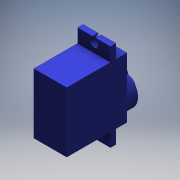
# Autodesk Inventor part: servo
Saved by Autodesk Inventor 2016 (Build 200138000, 138)
## iProperties
Created: 2017-12-28
Part Number: servo
Material: Genérico
Document SubType Name: Sheet Metal
Designer: David
Density: 1 g/cm^3
Sheet Metal Rule: Por defecto_mm
Appearance: Valor por defecto
Author: David
Autodesk Inventor part; units mm, degrees
ref_plane "YZ Plane" through (0, 0, 0) normal (1, 0, 0) x (0, 1, 0)
ref_plane "XZ Plane" through (0, 0, 0) normal (0, 1, 0) x (-1, 0, 0)
ref_plane "XY Plane" through (0, 0, 0) normal (0, 0, 1) x (1, 0, 0)
sketch "Boceto1" plane through (0, 0, 0) normal (0, 1, 0) x (-1, 0, 0)
  line L0 (0, 0) -> (12, 0)
  line L1 (12, 0) -> (12, -11)
  line L2 (12, -11) -> (0, -11)
  line L3 (0, -11) -> (0, 0)
  constraints: 8 end point, 2 parallel, 1 horizontal, 1 perpendicular
extrude "Extrusión1" add sketch "Boceto1" along normal blind 22
sketch "Boceto2" plane through (0, 0, -11) normal (0, 0, -1) x (-1, 0, 0)
  line L0 (12, 22) -> (0, 22) projected
  line L1 (0, 18) -> (12, 18)
  line L2 (0, 16) -> (12, 16)
  line L3 (12, 0) -> (12, 22) projected
  line L4 (0, 18) -> (0, 16)
  line L5 (0, 0) -> (0, 22) projected
  line L6 (12, 18) -> (12, 16)
  constraints: 8 end point, 2 collinear, 2 horizontal, 1 point on line
extrude "Extrusión2" add sketch "Boceto2" along normal blind 5 contours L3 L2 L4 L1
sketch "Boceto3" plane through (-12, 18, -11) normal (0, 1, 0) x (1, 0, 0)
  line L0 (0, 5) -> (12, 5) projected
  arc A0 (5.5, 4.5976) -> (6.5, 4.5976) centre (6, 3.1834) ccw
  line L1 (5.5, 4.5976) -> (5.5, 5)
  line L2 (5.5, 5) -> (6.5, 5)
  line L3 (6.5, 4.5976) -> (6.5, 5)
  point P0 (12, -11)
  constraints: 6 end point, 2 perpendicular, 2 point on circle, 2 point on line, 1 centre point
extrude "Extrusión3" cut sketch "Boceto3" against normal through all
mirror "Simetría1" about plane through (-12, 0, 0) normal (0, 0, 1) of "Extrusión1", "Extrusión2", "Extrusión3"
sketch "Boceto5" plane through (0, 22, 0) normal (0, 1, 0) x (1, 0, 0)
  line L0 (0, 11) -> (-12, 11) projected
  arc A0 (-3.6616, -0.5562) -> (-8.6574, -0.41) centre (-6, 4.9694) ccw
  arc A1 (-8.6574, -0.41) -> (-3.6616, -0.5562) centre (-6.1574, -0.412) ccw
  point P0 (0, 0)
  constraints: 4 point on circle, 2 centre point
extrude "Extrusión4" add sketch "Boceto5" along normal blind 4
sketch "Boceto6" plane through (0, 26, 0) normal (0, 1, 0) x (1, 0, 0)
  line L0 (0, 11) -> (0, 4.9694) projected
  arc A0 (0, 4.9694) -> (-12, 4.9694) centre (-6, 4.9694) ccw projected
  circle A1 centre (-6, 4.9694) radius 2
  point P0 (0, 0)
  constraints: 1 centre point, 1 coincident
extrude "Extrusión5" add sketch "Boceto6" along normal blind 3
equation "\"Radio_pliegue\" = Grosor"
equation "\"Anchura_desahogo_plegado\" = Grosor"
equation "\"Profundidad_desahogo_plegado\" = 0.5 * Grosor"
equation "\"Tamaño_destalonado\" = 4 * Grosor"
equation "\"Remanente_mínimo\" = 2 * Grosor"
equation "\"Radiodetransición\" = Radio_pliegue"
equation "\"Tamaño_de_radio_de_Jacobi\" = Radio_pliegue"
equation "\"TamañoSeparación\" = Grosor"
equation "\"Grosor\" = 0.5"
